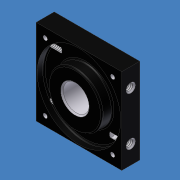
# Autodesk Inventor part: BB2-BackPlate
Saved by Autodesk Inventor 2012 (Build 160160000, 160)
## iProperties
Company: FirstCadLibrary
Shininess: 64.0
Length Units: 11269
Angle Units: 11279
Time Units: 11290
Mass Units: 11283
Length Display Precision: 3
Angle Display Precision: 2
Compacted: True
Part Number: BB2-BackPlate
Document SubType Name: Modeling
Created: 2007-01-08
Designer: Ed Sparks
Material: Aluminum-6061-AHC
Catalog Web Link: www.banebots.com
Vendor: BaneBots
Mass: 139.95 g
Surface Area: 166.186 cm^2
Volume: 51.6419 cm^3
Density: 2.71 g/cm^3
Density: 0.0
Volumn: 0.0
Area: 0.0
PropertySet Name: Model Information
Control State: 0
Master: False
Checked Out: False
Author: Ed Sparks
Autodesk Inventor part; units mm, degrees
ref_plane "YZ Plane" through (0, 0, 0) normal (1, 0, 0) x (0, 1, 0)
ref_plane "XZ Plane" through (0, 0, 0) normal (0, 1, 0) x (-1, 0, 0)
sketch "Sketch1" plane through (0, 0, 0) normal (0, 0, 1) x (1, 0, 0)
  line L0 (-31.75, 31.75) -> (31.75, 31.75)
  line L1 (31.75, 31.75) -> (31.75, -31.75)
  line L2 (31.75, -31.75) -> (-31.75, -31.75)
  line L3 (-31.75, -31.75) -> (-31.75, 31.75)
  line L4 (0, 0) -> (0, 31.75) construction
  line L5 (0, 0) -> (0, -31.75) construction
  line L6 (0, 0) -> (31.75, 0) construction
  line L7 (0, 0) -> (-31.75, 0) construction
  dimension "d0" = 63.5
  dimension "d1" = 63.5
  constraints: 16 end point, 4 midpoint, 2 collinear, 2 parallel, 1 horizontal, 1 perpendicular, 1 other
  measures "d0" distance of L0.end L1.end
  measures "d1" distance of L0.start L0.end
extrude "Extrusion1" add sketch "Sketch1" along normal mid plane 13.4
sketch "Sketch2" plane through (0, 0, 6.7) normal (0, 0, 1) x (1, 0, 0)
  circle A0 centre (0, 0) radius 31
  dimension "d4" = 62
  constraints: 1 centre point
  measures "d4" diameter of A0
extrude "Extrusion2" cut sketch "Sketch2" against normal blind 5
sketch "Sketch3" plane through (0, 0, 1.7) normal (0, 0, 1) x (1, 0, 0)
  circle A0 centre (-0.8072, 0) radius 20
  dimension "d7" = 40
  constraints: 1 centre point
  measures "d7" diameter of A0
extrude "Extrusion3" add sketch "Sketch3" along normal blind 8
fillet "Fillet1" radius 1 3 edges at (-20.8072, 0, 1.7) (-20.8072, 0, 9.7) (-31, 0, 1.7)
sketch "Sketch6" plane through (0, 0, -6.7) normal (0, 0, -1) x (-1, 0, 0)
  circle A0 centre (0, 0) radius 25
  dimension "d13" = 50
  constraints: 1 centre point
  measures "d13" diameter of A0
extrude "Extrusion4" add sketch "Sketch6" along normal blind 6
sketch "Sketch7" plane through (0, 0, -6.7) normal (0, 0, -1) x (-1, 0, 0)
  circle A0 centre (0, 0) radius 25 projected
  point P0 (-25, 25)
  dimension "d16" = 25
  dimension "d17" = 25
  measures "d16" horizontal distance of point (-25, 25) A0.centre
  measures "d17" horizontal distance of A0.centre point (-25, 25)
hole "Hole1" at (25, 25, -6.7) direction (0, 0, 1) diameter 3.2 end through all counterbore diameter 6.3 counterbore depth 10.3
pattern_circular "Circular Pattern1" count 4 over 360 about axis through (0, 0, -6.7) along (0, 0, -1) of "Hole1"
sketch "Sketch8" plane through (0, 0, -12.7) normal (0, 0, -1) x (-1, 0, 0)
  circle A0 centre (0, 0) radius 25 projected
  constraints: 1 coincident
hole "Hole2" at (0, 0, -12.7) direction (0, 0, 1) diameter 19.2 end through all
chamfer "Chamfer1" distance 1 angle 45 2 edges at (0, -9.6, 9.7) (0, -9.6, -12.7)
sketch "Sketch9" plane through (-31.75, -31.75, 6.7) normal (0, -1, 0) x (1, 0, 0)
  line L0 (63.5, 0) -> (0, 0) projected
  line L1 (0, 0) -> (0, -13.4) projected
  line L2 (0, -13.4) -> (63.5, -13.4) projected
  line L3 (63.5, 0) -> (63.5, -13.4) projected
  line L4 (0, -6.7) -> (63.5, -6.7) construction
  line L5 (31.75, 0) -> (31.75, -13.4) construction
  point P0 (13.75, -6.7)
  dimension "d37" = 18
  constraints: 4 end point, 4 midpoint, 1 point on line
  measures "d37" distance from line of point (13.75, -6.7) L5
hole "Hole3" at (-18, -31.75, 0) direction (0, 1, 0) diameter 4.978 depth 13.7 tip angle 118 thread size "1/4-20 UNC" class "1B" standard "ANSI Unified Screw Threads"
mirror "Mirror1" about plane through (0, 0, 0) normal (1, 0, 0) of "Hole3"
mirror "Mirror2" about plane through (0, 0, 0) normal (0, 1, 0) of "Hole3", "Mirror1"
chamfer "Chamfer2" distance 1 angle 45 4 edges at (-18, -31.75, 2.489) (18, -31.75, 2.489) (-18, 31.75, 2.489) (18, 31.75, 2.489)
ref_plane "Work Plane1" through (0, 25, 0) normal (0, 1, 0) x (-1, 0, 0)
sketch "Sketch10" plane through (0, 25, 0) normal (0, 1, 0) x (-1, 0, 0)
  line L0 (-31.75, -6.7) -> (31.75, -6.7) projected
  line L1 (0, -6.7) -> (0, -22.9157) construction
  point P0 (0, -10.2)
  dimension "d48" = 3.5
  constraints: 2 end point, 1 midpoint, 1 perpendicular, 1 point on line
  measures "d48" distance from line of point (0, -10.2) L0
hole "Hole4" at (0, 25, -10.2) direction (0, -1, 0) diameter 2.459 depth 7.5 tip angle 118 thread size "M3x0.5" class "6H" standard "ANSI Metric M Profile"
pattern_circular "Circular Pattern2" count 4 over 360 about axis through (0, 0, 79.8541) along (0, 0, -1) of "Hole4"
body "Solid1"
